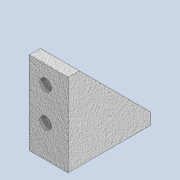
# Autodesk Inventor part: 2020 Extrusion 90deg 4Hole Aluminum Bracket
Saved by Autodesk Inventor 2022 (Build 260153000, 153)
## iProperties
Created: 2021-11-27
Part Number: 2020 Extrusion 90deg 4Hole Aluminum Bracket
Material: Generic
Document SubType Name: Modeling
Designer: Coy
Density: 1 g/cm^3
Appearance: Aluminum Cast
Author: Coy
Autodesk Inventor part; units mm, degrees
ref_plane "YZ Plane" through (0, 0, 0) normal (1, 0, 0) x (0, 1, 0)
ref_plane "XZ Plane" through (0, 0, 0) normal (0, 1, 0) x (-1, 0, 0)
ref_plane "XY Plane" through (0, 0, 0) normal (0, 0, 1) x (1, 0, 0)
sketch "Sketch1" plane through (0, 0, 0) normal (1, 0, 0) x (0, 1, 0)
  line L0 (0, 0) -> (0, -37.75)
  line L1 (0, -37.75) -> (5.15, -37.75)
  line L2 (5.15, -37.75) -> (37.75, -5.15)
  line L3 (37.75, -5.15) -> (37.75, 0)
  line L4 (37.75, 0) -> (0, 0)
  dimension "d0" = 135
  dimension "d1" = 37.75
  dimension "d2" = 5.15
  dimension "d3" = 5.15
  constraints: 10 end point, 2 perpendicular, 1 parallel, 1 vertical
  measures "d0" angle of L2 L1
  measures "d1" distance of L0.start L0.end
  measures "d2" distance of L0.end L1.end
  measures "d3" distance of L2.end L3.end
extrude "Extrusion1" add sketch "Sketch1" against normal blind 2.75
sketch "Sketch2" plane through (-2.75, 0, 0) normal (-1, 0, 0) x (0, 0, 1)
  line L0 (-37.75, 5.15) -> (-37.75, 0) projected
  line L1 (-37.75, 0) -> (0, 0) projected
  line L2 (0, 0) -> (0, 37.75) projected
  line L3 (0, 37.75) -> (-5.15, 37.75) projected
  line L4 (-5.15, 37.75) -> (-37.75, 5.15) projected
  line L5 (-37.75, 5.15) -> (-37.75, 0) projected
  line L6 (-37.75, 5.15) -> (-5.15, 5.15)
  line L7 (0, 37.75) -> (-5.15, 37.75) projected
  line L8 (-5.15, 5.15) -> (-5.15, 37.75)
  constraints: 4 end point, 1 perpendicular
extrude "Extrusion2" add sketch "Sketch2" along normal blind 15 contours L6 L8 L3 L2 L1 L0
sketch "Sketch3" plane through (-2.75, 5.15, -5.15) normal (0, 1, 0) x (1, 0, 0)
  line L0 (0, 0) -> (-15, 0) construction
  line L1 (-7.5, 0) -> (-7.5, 32.6) construction
  line L2 (2.75, 32.6) -> (-15, 32.6) construction
  circle A0 centre (-7.5, 24.475) radius 2.625
  circle A1 centre (-7.5, 9.475) radius 2.625
  point P0 (2.75, -5.15)
  dimension "d8" = 5.25
  dimension "d9" = 8.125
  dimension "d10" = 5.25
  dimension "d11" = 23.125
  constraints: 3 point on line, 2 centre point, 2 end point, 1 midpoint, 1 vertical
  measures "d8" diameter of A0
  measures "d9" distance of L1.end A0.centre
  measures "d10" diameter of A1
  measures "d11" distance from line of L2 A1.centre
extrude "Extrusion3" cut sketch "Sketch3" against normal up to next
sketch "Sketch4" plane through (-2.75, 5.15, -5.15) normal (0, 0, -1) x (-1, 0, 0)
  line L0 (0, 0) -> (15, 0) construction
  line L1 (7.5, 0) -> (7.5, 32.6) construction
  line L2 (0, 32.6) -> (15, 32.6) construction
  circle A0 centre (7.5, 24.475) radius 2.625
  circle A1 centre (7.5, 9.475) radius 2.625
  point P0 (-2.75, -5.15)
  dimension "d14" = 5.25
  dimension "d15" = 5.25
  dimension "d16" = 8.125
  dimension "d17" = 23.125
  constraints: 2 centre point, 2 end point, 2 midpoint, 2 point on line
  measures "d14" diameter of A0
  measures "d15" diameter of A1
  measures "d16" distance from line of L2 A0.centre
  measures "d17" distance from line of L2 A1.centre
extrude "Extrusion4" cut sketch "Sketch4" against normal up to next
equation "\"d3\" = d2"
equation "\"d10\" = d8"
equation "\"d15\" = d14"
body "Solid1"
